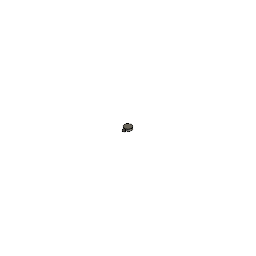
Catch_v2 (Autodesk Fusion 360 design; units mm, degrees)
Autodesk Fusion 360 part; units mm, degrees
sketch "Catch" plane through (0, 0, 0) normal (0, 0, 1) x (1, 0, 0)
  line L0 (-3.4202, 9.3969) -> (-5.1303, 14.0954) construction
  line L1 (3.4202, 9.3969) -> (5.1303, 14.0954) construction
  circle A0 centre (0, 0) radius 10 construction
  circle A1 centre (0, 0) radius 15 construction
  circle A2 centre (0, 0) radius 9
  circle A3 centre (0, 0) radius 13
  line L2 (-3.9731, 12.378) -> (-2.6036, 8.6152)
  line L3 (0, 0) -> (0, 15) construction
  line L4 (3.9731, 12.378) -> (2.6036, 8.6152)
  dimension "d119" = -1
  dimension "d120" = -2
  dimension "d121" = 0.5
  constraint coincident A3 L2.start
  constraint coincident A2 L2.end
  constraint parallel L0 L2
  constraint coincident A0.centre A1.centre
  constraint coincident A1 L3.end
  constraint vertical L3
  constraint symmetric L2.start L3 L4.start
  constraint symmetric L2.end L3 L4.end
  measures "d121" distance of L0 L2
extrude "Extrude6" add sketch "Catch" along normal blind 5.5 contours A2
extrude "Extrude7" add sketch "Catch" along normal blind 4 contours A2 A3 L2 L4 picked at (0, 11.65)
chamfer "Chamfer4" distance 4 angle 45 1 edges at (0, 13, 4) measured on face at (0, 11.65, 4)
move_body "Move2" bodies 1 to x (-1, 0, 0) y (0, -1, 0) z (0, 0, 1) at (0, 0, 0)
equation "d119 = -1 * Clearance"
equation "d120 = -1 * ( ( TailPieceOuter - TailPieceInner ) * 0.2 )"
equation "d121 = Clearance / 2"
equation "d122 = BodyBaseThickness + ( Clearance / 2 )"
equation "d124 = BodyBaseThickness - Clearance"
equation "d129 = BodyBaseThickness - Clearance"
equation "BodyBaseThickness = 5 mm"
equation "TailPieceInner = 20 mm"
equation "TailPieceOuter = 30 mm"
equation "Clearance = 1 mm"
named bodies: "Catch"
